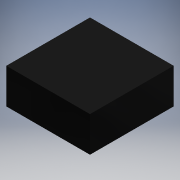
# Autodesk Inventor part: DC DC converter (M1730CQEA06065)
Saved by Autodesk Inventor 2017 (Build 210142000, 142)
## iProperties
Part Number: DC DC converter (M1730CQEA06065)
Material: Generisch
Document SubType Name: Modeling
Designer: ExCISS
Density: 1 g/cm^3
Appearance: Vorgabe
Author: ExCISS
Autodesk Inventor part; units mm, degrees
ref_plane "YZ Plane" through (0, 0, 0) normal (1, 0, 0) x (0, 1, 0)
ref_plane "XZ Plane" through (0, 0, 0) normal (0, 1, 0) x (-1, 0, 0)
ref_plane "XY Plane" through (0, 0, 0) normal (0, 0, 1) x (1, 0, 0)
sketch "Skizze1" plane through (0, 0, 0) normal (0, 0, 1) x (1, 0, 0)
  line L0 (-19.05, 19.05) -> (19.05, 19.05)
  line L1 (19.05, 19.05) -> (19.05, -19.05)
  line L2 (19.05, -19.05) -> (-19.05, -19.05)
  line L3 (-19.05, -19.05) -> (-19.05, 19.05)
  line L4 (-19.05, 19.05) -> (19.05, -19.05) construction
  point P0 (0, 0)
  point P1 (0, 0)
  dimension "d0" = 38.1
  dimension "d1" = 38.1
  constraints: 10 end point, 2 parallel, 1 coincident, 1 horizontal, 1 midpoint, 1 perpendicular
  measures "d0" distance of L1.end L2.end
  measures "d1" distance of L0.end L1.end
extrude "Extrusion1" add sketch "Skizze1" along normal mid plane 16
sketch "Skizze2" plane through (0, 0, -8) normal (0, 0, -1) x (-1, 0, 0)
  line L0 (19.05, 19.05) -> (-19.05, 19.05) construction
  line L1 (-19.05, 19.05) -> (-19.05, -19.05) construction
  line L2 (-19.05, -19.05) -> (19.05, -19.05) construction
  line L3 (19.05, -19.05) -> (19.05, 19.05) construction
  line L4 (-19.05, -19.05) -> (-19.05, 19.05) construction
  line L5 (-19.05, -19.05) -> (-19.05, -15.24) construction
  line L6 (19.05, -19.05) -> (-19.05, -19.05) construction
  line L7 (19.05, -19.05) -> (19.05, -15.24) construction
  line L8 (19.05, 19.05) -> (19.05, -19.05) construction
  line L9 (-19.05, -15.24) -> (-10.16, -15.24) construction
  line L10 (19.05, -15.24) -> (10.16, -15.24) construction
  line L11 (-19.05, 19.05) -> (19.05, 19.05) construction
  line L12 (-19.05, 19.05) -> (-19.05, 15.24) construction
  line L13 (-19.05, 15.24) -> (-12.7, 15.24) construction
  line L14 (19.05, 19.05) -> (19.05, 15.24) construction
  line L15 (19.05, 15.24) -> (12.7, 15.24) construction
  circle A0 centre (-10.16, -15.24) radius 0.395
  circle A1 centre (-12.7, 15.24) radius 0.395
  circle A2 centre (12.7, 15.24) radius 0.395
  circle A3 centre (10.16, -15.24) radius 0.395
  point P0 (0, 0)
  dimension "d4" = 3.81
  dimension "d5" = 3.81
  dimension "d8" = 8.89
  dimension "d9" = 8.89
  dimension "d10" = 3.81
  dimension "d11" = 6.35
  dimension "d12" = 3.81
  dimension "d13" = 6.35
  dimension "d14" = 0.79
  dimension "d15" = 0.79
  dimension "d16" = 0.79
  dimension "d17" = 0.79
  constraints: 16 end point, 8 coincident, 4 centre point, 4 point on line, 3 perpendicular, 1 horizontal
  measures "d4" distance of L1.end L5.end
  measures "d5" distance of L2.end L7.end
  measures "d8" distance of L5.end L9.end
  measures "d9" distance of L7.end L10.end
  measures "d10" distance of L0.end L12.end
  measures "d11" distance of L12.end L13.end
  measures "d12" distance of L0.start L14.end
  measures "d13" distance of L14.end L15.end
  measures "d14" diameter of A0
  measures "d15" diameter of A1
  measures "d16" diameter of A2
  measures "d17" diameter of A3
extrude "Extrusion4" add sketch "Skizze2" along normal blind 5.08
sketch "Skizze3" plane through (10.16, -15.24, -13.08) normal (0, 0, -1) x (-1, 0, 0)
  circle A0 centre (0, 0) radius 0.395 projected
  circle A1 centre (20.32, 0) radius 0.395 projected
  circle A2 centre (22.86, 30.48) radius 0.395 projected
  circle A3 centre (-2.54, 30.48) radius 0.395 projected
  point P0 (10.16, 15.24)
extrude "Extrusion5" cut sketch "Skizze3" against normal blind 2
